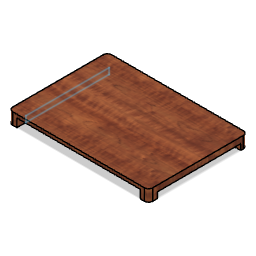
plateau-jeu-bois-c-ache v2 (Autodesk Fusion 360 design; units mm, degrees)
Autodesk Fusion 360 part; units mm, degrees
sketch "Esquisse1" plane through (0, 0, 0) normal (0, 1, 0) x (1, 0, 0)
  line L0 (-50, 50) -> (791, 50)
  line L1 (791, 50) -> (791, -544)
  line L2 (791, -544) -> (-50, -544)
  line L3 (-50, -544) -> (-50, 50)
  dimension "d1" = 594
  dimension "d2" = 841
  constraint horizontal L0
  constraint vertical L1
  constraint horizontal L2
  constraint vertical L3
  measures "d1" distance of L0.end L1.end
  measures "d2" distance of L0.start L0.end
extrude "Extrusion1" add sketch "Esquisse1" along normal blind 20
sketch "Esquisse3" plane through (0, 0, 0) normal (0, 1, 0) x (1, 0, 0)
  line L0 (-50, -544) -> (0, -544)
  line L1 (0, -544) -> (0, 50)
  line L2 (0, 50) -> (-50, 50)
  line L3 (-50, 50) -> (-50, -544)
  line L4 (741, -544) -> (791, -544)
  line L5 (791, -544) -> (791, 50)
  line L6 (791, 50) -> (741, 50)
  line L7 (741, 50) -> (741, -544)
  point P0 (-50, -544)
  point P1 (791, -544)
  point P2 (-25, -247)
  point P3 (766, -247)
  dimension "d7" = 50
  dimension "d8" = 594
  dimension "d9" = 50
  dimension "d10" = 594
  constraint horizontal L0
  constraint vertical L1
  constraint horizontal L2
  constraint vertical L3
  constraint coincident P0 L0.start
  constraint horizontal L4
  constraint vertical L5
  constraint horizontal L6
  constraint vertical L7
  constraint coincident P1 L4.end
  measures "d7" distance of P0 L0.end
  measures "d8" distance of P0 L2.end
  measures "d9" distance of L4.start P1
  measures "d10" distance of P1 L5.end
extrude "Extrusion2" add sketch "Esquisse3" against normal blind 50
sketch "Esquisse8" plane through (0, 0, 0) normal (1, 0, 0) x (0, 0, -1)
  line L0 (-490, -15) -> (10, -15)
  line L1 (10, -15) -> (10, -50)
  line L2 (10, -50) -> (-490, -50)
  line L3 (-490, -50) -> (-490, -15)
  dimension "d17" = 35
  dimension "d18" = 500
  constraint horizontal L0
  constraint vertical L1
  constraint horizontal L2
  constraint vertical L3
  measures "d17" distance of L0.start L2.end
  measures "d18" distance of L0.start L0.end
extrude "Extrusion3" cut sketch "Esquisse8" along normal mid plane 1850
fillet "Congé1" radius 25 4 edges at (-50, -15, 544) (-50, -15, -50) (791, -15, 544) (791, -15, -50)
named bodies: "Plateau"
